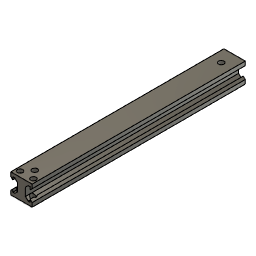
Направляющая рейка v5 (Autodesk Fusion 360 design; units mm, degrees)
Autodesk Fusion 360 part; units mm, degrees
sketch "Sketch1" plane through (0, 0, 0) normal (1, 0, 0) x (0, 0, -1)
  line L0 (-150, 0) -> (-150, 10)
  line L1 (-150, 10) -> (0, 10)
  line L2 (0, 10) -> (0, 0)
  line L3 (-150, 10) -> (-140, 10)
  line L4 (-140, 10) -> (-140, 0)
  line L5 (-140, 0) -> (-150, 0)
  line L6 (-150, 0) -> (-150, 10)
  line L7 (0, 0) -> (-10, 0)
  line L8 (-10, 0) -> (-10, 10)
  line L9 (-10, 10) -> (0, 10)
  line L10 (0, 10) -> (0, 0)
  line L11 (-2.5, 0) -> (-12.5, 0)
  line L12 (-12.5, 10) -> (-2.5, 10)
  line L13 (-150, 0) -> (-147.5, 0)
  line L14 (0, 0) -> (-147.5, 0)
  dimension "d2" = 10
  dimension "d3" = 130
  dimension "d4" = 10
  dimension "d9" = 10
  dimension "d11" = 10
  constraint horizontal L14
  constraint vertical L0
  constraint horizontal L1
  constraint vertical L2
  constraint coincident L2.end L7.start
  constraint horizontal L3
  constraint vertical L4
  constraint horizontal L5
  constraint vertical L6
  constraint coincident L4.end L14
  constraint horizontal L7
  constraint vertical L8
  constraint horizontal L9
  constraint vertical L10
  constraint coincident L1 L8.end
  constraint horizontal L11
  constraint parallel L11 L12
  constraint coincident L1 L12.end
  measures "d2" distance of L2.end L1.end
  measures "d3" distance of L4 L8
  measures "d4" distance of L0 L4
  measures "d9" distance of L8.end L1.end
  measures "d11" distance of L11.end L12.start
extrude "Extrude1" add sketch "Sketch1" along normal blind 15
extrude "Extrude4" add 1 faces at (15, 3.3333, 55) along direction (1, 0, 0) blind 10
extrude "Extrude5" add 1 faces at (8.3333, 10, 100) along direction (0, 1, 0) blind 5
sketch "Sketch2" plane through (0, 0, 0) normal (0, 0, -1) x (-1, 0, 0)
  line L0 (0, 15) -> (-25, 15)
  line L1 (-25, 15) -> (-25, 0)
  line L2 (-25, 0) -> (0, 0)
  line L3 (-25, 0) -> (-25, 3)
  line L4 (-25, 15) -> (-25, 12)
  line L5 (-23.5, 10.5) -> (-25, 12)
  line L6 (-23.5, 4.5) -> (-25, 3)
  line L7 (-23.5, 4.5) -> (-23.5, 2.5)
  line L8 (-23.5, 12.5) -> (-22, 12.5)
  line L9 (-23.5, 2.5) -> (-22, 2.5)
  line L10 (-22, 2.5) -> (-20, 4.5)
  line L11 (-20, 4.5) -> (-20, 10.5)
  line L12 (-20, 10.5) -> (-22, 12.5)
  line L13 (-23.5, 2.5) -> (-23.5, 4.5)
  line L14 (-23.5, 10.5) -> (-23.5, 12.5)
  line L15 (-20, 4.5) -> (-14, 4.5)
  line L16 (-14, 4.5) -> (-14, 10.5)
  line L17 (-14, 10.5) -> (-20, 10.5)
  line L18 (-20, 10.5) -> (-20, 4.5)
  line L19 (-17, 4.5) -> (-17, 10.5)
  line L20 (-14, 7.5) -> (-20, 7.5)
  line L21 (-10.5, 4.5) -> (-9, 3)
  line L22 (-10.5, 2.5) -> (-10.5, 4.5)
  line L23 (-10.5, 2.5) -> (-12, 2.5)
  line L24 (-12, 2.5) -> (-14, 4.5)
  line L25 (-14, 4.5) -> (-14, 10.5)
  line L26 (-14, 10.5) -> (-12, 12.5)
  line L27 (-10.5, 12.5) -> (-12, 12.5)
  line L28 (-10.5, 10.5) -> (-10.5, 12.5)
  line L29 (-10.5, 10.5) -> (-9, 12)
  line L30 (-9, 3) -> (-9, 12)
  line L31 (-9, 0) -> (-25, 0)
  line L32 (-25, 0) -> (-25, 15)
  line L33 (-25, 15) -> (-9, 15)
  line L34 (-9, 15) -> (-9, 0)
  line L35 (0, 0) -> (-15, 0)
  line L36 (-15, 0) -> (-15, 15)
  line L37 (-15, 15) -> (0, 15)
  line L38 (0, 15) -> (0, 0)
  line L39 (0, 0) -> (0, 15)
  dimension "d22" = 3
  dimension "d23" = 3
  dimension "d24" = 6
  dimension "d27" = 10
  dimension "d28" = 6
  dimension "d29" = 135
  dimension "d30" = 135
  dimension "d31" = 45
  dimension "d32" = 45.001
  dimension "d33" = 1.5
  dimension "d34" = 1.5
  dimension "d35" = 2.1213
  dimension "d37" = 2
  dimension "d38" = 6
  dimension "d39" = 6
  dimension "d40" = 16
  dimension "d45" = 15
  dimension "d48" = 15
  constraint coincident L1.end L2.start
  constraint perpendicular L0 L3
  constraint coincident L0.end L1.start
  constraint perpendicular L0 L4
  constraint perpendicular L8 L13
  constraint perpendicular L7 L9
  constraint perpendicular L8 L11
  constraint collinear L13 L14
  constraint horizontal L15
  constraint vertical L16
  constraint horizontal L17
  constraint vertical L18
  constraint midpoint L15 L19.start
  constraint midpoint L17 L19.end
  constraint midpoint L16 L20.start
  constraint midpoint L18 L20.end
  constraint symmetric L3.end L19 L21.end
  constraint symmetric L4.end L19 L29.end
  constraint symmetric L6.start L19 L21.start
  constraint symmetric L5.start L19 L28.start
  constraint symmetric L7.end L19 L22.start
  constraint symmetric L8.start L19 L27.start
  constraint symmetric L8.end L19 L26.end
  constraint symmetric L9.end L19 L23.end
  constraint symmetric L10.end L19 L15.end
  constraint symmetric L11.end L19 L16.end
  constraint horizontal L31
  constraint vertical L32
  constraint horizontal L33
  constraint vertical L34
  constraint coincident L2 L31.start
  constraint horizontal L35
  constraint vertical L36
  constraint horizontal L37
  constraint vertical L38
  constraint coincident L2.end L35.start
  measures "d22" distance of L1.end L3.end
  measures "d23" distance of L0.end L4.end
  measures "d24" distance of L6.start L5.start
  measures "d27" distance of L7.end L8.start
  measures "d28" distance of L10.end L11.end
  measures "d29" angle of L11 L12
  measures "d30" angle of L10 L11
  measures "d31" angle of L6 L7
  measures "d32" angle of L5 L14
  measures "d33" distance of L7.end L9.end
  measures "d34" distance of L8.start L8.end
  measures "d35" distance of L4.end L5.start
  measures "d37" distance of L6.start L7.end
  measures "d38" distance of L10.end L15.end
  measures "d39" distance of L10.end L11.end
  measures "d40" distance of L32 L34
  measures "d45" distance of L2.end L35.end
  measures "d48" distance of L35 L37
extrude "Extrude6" cut sketch "Sketch2" against normal blind 185 contours L16 L21 L22 L23 L24 L25 L26 L27 L28 L29 L30 L34 | L1 L5 L6 L7 L8 L9 L10 L11 L12 L13 L14 L18 L32
extrude "Extrude8" add sketch "Sketch2" along normal blind 10 contours L0 L17 L26 L27 L28 L29 L33 L34 L36 L37 | L0 L1 L4 L5 L8 L12 L14 L17 L32 L33 L36 | L2 L15 L21 L22 L23 L24 L31 L34 L35 L36 | L17 L19 L20 L36 | L16 L17 L20 L25 L36 | L1 L2 L3 L6 L7 L9 L10 L13 L15 L31 L32 L36 | L11 L17 L18 L19 L20 | L15 L19 L20 L36 | L15 L16 L20 L25 L36 | L11 L15 L18 L19 L20
extrude "Extrude9" cut 1 faces at (3, 6, 0) along direction (0, 0, 1) blind 240
sketch "Sketch3" plane through (0, 0, 0) normal (0, -1, 0) x (1, 0, 0)
  line L0 (9, 150) -> (9, -10)
  line L1 (9, -10) -> (25, -10)
  line L2 (25, -10) -> (25, 150)
  line L3 (25, 150) -> (9, 150)
  line L4 (25, 150) -> (25, 145)
  line L5 (25, 145) -> (9, 145)
  line L6 (9, 145) -> (9, -5)
  line L7 (9, -5) -> (25, -5)
  line L8 (25, -5) -> (25, 145)
  line L9 (25, 145) -> (9, 145)
  line L10 (9, 145) -> (9, 135)
  line L11 (9, 135) -> (25, 135)
  line L12 (25, 135) -> (25, 145)
  line L13 (9, -5) -> (25, -5)
  line L14 (25, -5) -> (25, 5)
  line L15 (25, 5) -> (9, 5)
  line L16 (9, 5) -> (9, -5)
  circle A0 centre (17, -0.0404) radius 2
  circle A1 centre (17, 140) radius 2
  dimension "d51" = 16
  dimension "d52" = 150
  dimension "d53" = 5
  dimension "d54" = 10
  dimension "d55" = 130
  dimension "d56" = 16
  dimension "d63" = 4
  dimension "d64" = 4
  dimension "d65" = 140.0404
  constraint coincident L2.end L3.start
  constraint coincident L2 L4.end
  constraint perpendicular L3 L4
  constraint horizontal L5
  constraint vertical L6
  constraint horizontal L7
  constraint vertical L8
  constraint horizontal L9
  constraint vertical L10
  constraint horizontal L11
  constraint vertical L12
  constraint horizontal L13
  constraint vertical L14
  constraint horizontal L15
  constraint vertical L16
  constraint coincident L8 L14.end
  measures "d51" distance of L4.end L5.end
  measures "d52" distance of L4.end L7.end
  measures "d53" distance of L3 L5
  measures "d54" distance of L4.end L11.end
  measures "d55" distance of L11 L15
  measures "d56" distance of L10 L12
  measures "d63" diameter of A0
  measures "d64" diameter of A1
  measures "d65" distance of A0.centre A1.centre
extrude "Extrude10" cut sketch "Sketch3" against normal blind 50 contours A0 | A1
sketch "Sketch4" plane through (0, 15, 0) normal (0, 1, 0) x (-1, 0, 0)
  circle A0 centre (-17, 140) radius 2
  circle A1 centre (-17, -0.0404) radius 2
  line L0 (-9, -10) -> (-9, 150)
  line L1 (-9, 150) -> (-25, 150)
  line L2 (-25, 150) -> (-25, -10)
  line L3 (-25, -10) -> (-9, -10)
  circle A2 centre (-12, 146) radius 2
  circle A3 centre (-22, 146) radius 2
  dimension "d66" = 4
  dimension "d68" = 4
  dimension "d69" = 3
  dimension "d70" = 3
  dimension "d71" = 4
  dimension "d72" = 4
  measures "d66" diameter of A2
  measures "d68" diameter of A3
  measures "d69" distance of L0 A2.centre
  measures "d70" distance of L2 A3.centre
  measures "d71" distance of L1 A3.centre
  measures "d72" distance of L1 A2.centre
extrude "Extrude11" cut sketch "Sketch4" against normal blind 24 contours A2 | A3
